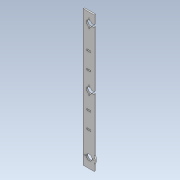
# Autodesk Inventor part: chassis_1_1_3
Saved by Autodesk Inventor 2022 (Build 260153000, 153)
## iProperties
Created: 2023-04-21
Part Number: chassis_1_1_3
Material: 一般
Document SubType Name: Modeling
Designer: JOU
Density: 1 g/cm^3
Appearance: 預設
Author: JOU
Autodesk Inventor part; units mm, degrees
ref_plane "YZ Plane" through (0, 0, 0) normal (1, 0, 0) x (0, 1, 0)
ref_plane "XZ Plane" through (0, 0, 0) normal (0, 1, 0) x (-1, 0, 0)
ref_plane "XY Plane" through (0, 0, 0) normal (0, 0, 1) x (1, 0, 0)
sketch "草圖1" plane through (0, 0, 0) normal (0, 0, 1) x (1, 0, 0)
  line L0 (-6, 142.5) -> (-10.5456, 142.5)
  arc A0 (-10.5456, 147.5) -> (-10.5456, 142.5) centre (-16, 145) ccw
  line L1 (-10.5456, 147.5) -> (-6, 147.5)
  circle A1 centre (-16, 153.5) radius 1.5
  circle A2 centre (-16, 136.5) radius 1.5
  circle A3 centre (-16, 275) radius 1.5
  circle A4 centre (-16, 258) radius 1.5
  circle A5 centre (-16, 23.5) radius 6
  circle A6 centre (-24.5, 23.5) radius 1.5
  circle A7 centre (-7.5, 23.5) radius 1.5
  line L2 (-6, 3) -> (-6, 16)
  line L3 (-6, 31) -> (-6, 142.5)
  arc A8 (-6, 16) -> (-6, 31) centre (-16, 23.5) ccw
  line L4 (-28.5, 3) -> (-28.5, 287)
  arc A9 (-10.546, 269.0008) -> (-10.546, 263.9992) centre (-16, 266.5) ccw
  line L5 (-28.5, 3) -> (-6, 3)
  line L6 (-6, 287) -> (-28.5, 287)
  line L7 (-6, 269.0008) -> (-10.546, 269.0008)
  line L8 (-10.546, 263.9992) -> (-6, 263.9992)
  line L9 (-6, 147.5) -> (-6, 263.9992)
  line L10 (-6, 269.0008) -> (-6, 287)
  circle A10 centre (-16, 23.5) radius 12.5 construction
  line L11 (-21, 72.05) -> (-6, 72.05)
  line L12 (-6, 72.05) -> (-6, 75)
  line L13 (-6, 75) -> (-21, 75)
  line L14 (-21, 75) -> (-21, 72.05)
  line L15 (-6, 107.05) -> (-21, 107.05)
  line L16 (-21, 107.05) -> (-21, 110)
  line L17 (-21, 110) -> (-6, 110)
  line L18 (-6, 110) -> (-6, 107.05)
  line L19 (-6, 180) -> (-21, 180)
  line L20 (-21, 180) -> (-21, 182.95)
  line L21 (-21, 182.95) -> (-6, 182.95)
  line L22 (-6, 182.95) -> (-6, 180)
  line L23 (-6, 215) -> (-21, 215)
  line L24 (-21, 215) -> (-21, 217.95)
  line L25 (-21, 217.95) -> (-6, 217.95)
  line L26 (-6, 217.95) -> (-6, 215)
  line L27 (-13, 217.95) -> (-13, 215)
  line L28 (-13, 182.95) -> (-13, 180)
  line L29 (-13, 110) -> (-13, 107.05)
  line L30 (-13, 75) -> (-13, 72.05)
  point P0 (0, 0)
  point P1 (0, 0)
  point P2 (-6, 110)
  dimension "d0" = 12
  dimension "d3" = 3
  dimension "d4" = 12
  dimension "d5" = 10
  dimension "d6" = 12.5
  dimension "d9" = 8.5
  dimension "d10" = 8.5
  dimension "d12" = 20.5
  dimension "d13" = 4.546
  dimension "d14" = 5.0015
  dimension "d17" = 2.95
  dimension "d18" = 2.95
  dimension "d19" = 2.95
  dimension "d20" = 2.95
  dimension "d21" = 7.5
  dimension "d22" = 35
  dimension "d23" = 70
  dimension "d24" = 35
  dimension "d25" = 70
  dimension "d26" = 8
  constraints: 62 end point, 21 point on line, 10 centre point, 9 horizontal, 9 parallel, 6 point on circle, 5 perpendicular, 5 vertical, 2 coincident, 2 horizontal alignment, 1 equal radius, 22 other
  measures "d0" diameter of A5
  measures "d3" diameter of A6
  measures "d4" diameter of A9
  measures "d5" distance from line of L2 A8.centre
  measures "d6" radius of A8
  measures "d9" distance of A8.centre A6.centre
  measures "d10" distance of A8.centre A7.centre
  measures "d12" distance from line of A5.centre L5
  measures "d13" distance of L8.start L8.end
  measures "d14" distance between parallel lines of L8 L7
  measures "d17" distance of L13.end L11.start
  measures "d18" distance of L15.end L16.end
  measures "d19" distance of L19.end L20.end
  measures "d20" distance of L23.end L24.end
  measures "d21" distance between parallel lines of L4 L20
  measures "d22" distance from line of A0.centre L17
  measures "d23" distance from line of L13 A0.centre
  measures "d24" distance from line of L19 A0.centre
  measures "d25" distance from line of L23 A0.centre
  measures "d26" distance between parallel lines of L28 L20
extrude "擠出1" add sketch "草圖1" along normal blind 3 contours L3 L17 L16 L15 L13 L14 L11 A8 L2 L5 L4 L6 L10 L7 A9 L8 L9 L25 L24 L23 L21 L20 L19 L1 A0 L0 | L3 L15 L29 L17 | L3 L11 L30 L13 | L19 L28 L21 L9 | L23 L27 L25 L9
